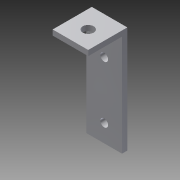
# Autodesk Inventor part: Servo catch front
Saved by Autodesk Inventor 2015 (Build 190159000, 159)
## iProperties
Created: 2015-05-18
Part Number: Servo catch front
Material: アルミニウム 1100-H14
Document SubType Name: Modeling
Designer: kenta
Density: 2.7 g/cm^3
Appearance: サテン
Mass: 1.53839 g
Surface Area: 9.43542 cm^2
Volume: 0.569775 cm^3
Author: kenta
Autodesk Inventor part; units mm, degrees
ref_plane "YZ Plane" through (0, 0, 0) normal (1, 0, 0) x (0, 1, 0)
ref_plane "XZ Plane" through (0, 0, 0) normal (0, 1, 0) x (-1, 0, 0)
ref_plane "XY Plane" through (0, 0, 0) normal (0, 0, 1) x (1, 0, 0)
sketch "スケッチ1" plane through (0, 0, 0) normal (0, 0, 1) x (1, 0, 0)
  line L0 (-5, 5) -> (5, 5)
  line L1 (5, 5) -> (5, -5)
  line L2 (5, -5) -> (-5, -5)
  line L3 (-5, -5) -> (-5, 5)
  line L4 (-5, 5) -> (5, -5) construction
  line L5 (5, 5) -> (-5, -5) construction
  point P0 (0, 0)
  dimension "d0" = 10
  dimension "d1" = 10
  constraints: 12 end point, 2 midpoint, 2 parallel, 1 horizontal, 1 perpendicular
  measures "d0" distance of L1.end L2.end
  measures "d1" distance of L0.end L1.end
extrude "押し出し1" add sketch "スケッチ1" along normal blind 1
sketch "スケッチ4" plane through (0, 0, 1) normal (0, 0, 1) x (1, 0, 0)
  line L0 (-5, 5) -> (5, 5)
  line L1 (5, 5) -> (5, 6)
  line L2 (5, 6) -> (-5, 6)
  line L3 (-5, 6) -> (-5, 5)
  point P0 (0, 0)
  dimension "d11" = 1
  constraints: 8 end point, 2 parallel, 1 horizontal, 1 perpendicular
  measures "d11" distance of L1.end L0.end
extrude "押し出し2" add sketch "スケッチ4" against normal blind 30
sketch "スケッチ9" plane through (0, 0, 0) normal (0, 0, -1) x (-1, 0, 0)
  line L0 (-5, -5) -> (5, -5)
  line L1 (5, -5) -> (5, 5)
  line L2 (5, 5) -> (-5, 5)
  line L3 (-5, 5) -> (-5, -5)
  point P0 (0, 0)
  constraints: 8 end point, 2 parallel, 1 horizontal, 1 perpendicular
extrude "押し出し6" add sketch "スケッチ9" along normal blind 0.5
sketch "スケッチ10" plane through (0, 0, 1) normal (0, 0, 1) x (1, 0, 0)
  circle A0 centre (0, 0) radius 1.55
  dimension "d37" = 3.1
  constraints: 1 centre point
  measures "d37" diameter of A0
extrude "押し出し7" cut sketch "スケッチ10" against normal blind 3
sketch "スケッチ11" plane through (-5, 5, -29) normal (0, -1, 0) x (1, 0, 0)
  line L0 (0, 0) -> (10, 0)
  line L1 (10, 0) -> (10, 28.5)
  line L2 (10, 28.5) -> (0, 28.5)
  line L3 (0, 28.5) -> (0, 0)
  point P0 (5, 29)
  constraints: 8 end point, 2 parallel, 1 horizontal, 1 perpendicular
extrude "押し出し8" add sketch "スケッチ11" along normal blind 0.5
sketch "スケッチ12" plane through (-5, 6, 1) normal (0, 1, 0) x (1, 0, 0)
  line L0 (10, 0) -> (10, 30) projected
  point P0 (5, 1)
  point P1 (5, 25)
  point P2 (5, 9)
  dimension "d42" = 16
  dimension "d43" = 8
  dimension "d44" = 5
  measures "d42" distance of point (5, 9) point (5, 25)
  measures "d43" distance of point (5, 9) point (5, 1)
  measures "d44" distance from line of point (5, 25) L0
hole "穴3" at (0, 6, -24) at (0, 6, -8) direction (0, -1, 0) diameter 2.2 depth 8 tip angle 118
